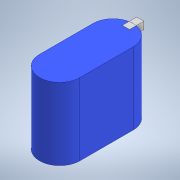
# Autodesk Inventor part: battery
Saved by Autodesk Inventor 2020 (Build 240168000, 168)
## iProperties
Created: 2019-09-19
Part Number: battery
Material: Generic
Document SubType Name: Modeling
Designer: suchanek
Density: 1 g/cm^3
Appearance: Default
Author: suchanek
Autodesk Inventor part; units mm, degrees
ref_plane "YZ Plane" through (0, 0, 0) normal (1, 0, 0) x (0, 1, 0)
ref_plane "XZ Plane" through (0, 0, 0) normal (0, 1, 0) x (-1, 0, 0)
ref_plane "XY Plane" through (0, 0, 0) normal (0, 0, 1) x (1, 0, 0)
sketch "Sketch1" plane through (0, 0, 0) normal (0, 1, 0) x (-1, 0, 0)
  line L0 (0, 65) -> (0, 0) construction
  line L1 (-14, 51) -> (-14, 14)
  line L2 (14, 14) -> (14, 51)
  arc A0 (14, 51) -> (-14, 51) centre (0, 51) ccw
  arc A1 (-14, 14) -> (14, 14) centre (0, 14) ccw
  point P0 (0, 32.5)
  dimension "d0" = 65
  dimension "d1" = 28
  constraints: 8 end point, 6 point on circle, 4 tangent, 2 centre point, 2 point on line, 1 midpoint, 1 parallel, 1 vertical
  measures "d0" distance of L0.end L0.start
  measures "d1" distance between parallel lines of L1 L2
extrude "Extrusion1" add sketch "Sketch1" along normal blind 50
sketch "Sketch2" plane through (0, 50, 0) normal (0, 1, 0) x (1, 0, 0)
  line L0 (-2.5878, -5) -> (2.4122, -5)
  line L1 (2.4122, -5) -> (2.4122, 5)
  line L2 (2.4122, 5) -> (-2.5878, 5)
  line L3 (-2.5878, 5) -> (-2.5878, -5)
  point P0 (0, 0)
  dimension "d4" = 5
  dimension "d5" = 10
  dimension "d6" = 5
  constraints: 8 end point, 2 parallel, 1 horizontal, 1 perpendicular
  measures "d4" distance of L2.end L1.end
  measures "d5" distance of L1.end L0.end
  measures "d6" distance from line of L2 point (0, 0)
extrude "Extrusion2" add sketch "Sketch2" along normal blind 0.1 and the other way blind 5 separate body
body "Solid1"
body "Solid2"
